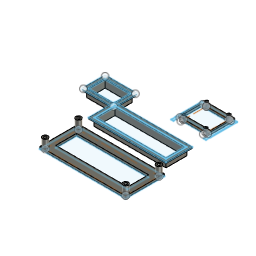
bayesCalc-oled-frame v13 (Autodesk Fusion 360 design; units mm, degrees)
Autodesk Fusion 360 part; units mm, degrees
note: some values were not read from the file. Set by a fixed rule: which sketch regions a step uses.
sketch "Sketch1" plane through (0, 0, 0) normal (0, 0, 1) x (1, 0, 0)
  line L0 (-26.7, -2.5) -> (-1.5, -2.5)
  line L1 (-1.5, -2.5) -> (-1.5, -19.7)
  line L2 (-1.5, -19.7) -> (-26.7, -19.7)
  line L3 (-26.7, -19.7) -> (-26.7, -2.5)
  line L4 (-2.5, -18.7) -> (-25.7, -18.7)
  line L5 (-25.7, -18.7) -> (-25.7, -3.5)
  line L6 (-25.7, -3.5) -> (-2.5, -3.5)
  line L7 (-2.5, -3.5) -> (-2.5, -18.7)
  line L8 (-29.2, -21.2) -> (-29.2, -1)
  line L9 (-28.2, 0) -> (0, 0)
  line L10 (1, -1) -> (1, -21.2)
  line L11 (0, -22.2) -> (-28.2, -22.2)
  arc A0 (1, -1) -> (0, 0) centre (0, -1) ccw
  arc A1 (0, -22.2) -> (1, -21.2) centre (0, -21.2) ccw
  arc A2 (-28.2, 0) -> (-29.2, -1) centre (-28.2, -1) ccw
  arc A3 (-29.2, -21.2) -> (-28.2, -22.2) centre (-28.2, -21.2) ccw
  dimension "d1" = 25.2
  dimension "d2" = 17.2
  dimension "d3" = 1
  dimension "d36" = 1
  dimension "d37" = 1
  dimension "d50" = 2.5
  dimension "d51" = 2.5
  dimension "d52" = 2.5
  dimension "d53" = 2.5
  constraint horizontal L0
  constraint vertical L1
  constraint horizontal L2
  constraint vertical L3
  constraint parallel L3 L8
  constraint parallel L0 L9
  constraint parallel L1 L10
  constraint parallel L2 L11
  constraint tangent L9 A0
  constraint tangent L10 A0
  constraint tangent L10 A1
  constraint tangent L11 A1
  constraint tangent L8 A2
  constraint tangent L9 A2
  constraint equal A1 A2
  constraint tangent L8 A3
  constraint tangent L11 A3
  constraint equal A1 A3
  measures "d1" distance of L0.start L0.end
  measures "d2" distance of L0.start L2.end
  measures "d36" radius of A0
  measures "d37" radius of A1
  measures "d50" distance of L2 L11
  measures "d51" distance of L0 L9
  measures "d52" distance of L3 L8
  measures "d53" distance of L1 L10
extrude "Extrude1" add sketch "Sketch1" against normal blind 7 contours L0 L1 L2 L3 makes body 1
extrude "Extrude2" add sketch "Sketch1" against normal blind 1 separate body contours L8 L9 L10 L11 A0 A1 A2 A3 makes body 2
sketch "Sketch2" plane through (0, 0, 0) normal (0, 0, 1) x (1, 0, 0)
  line L0 (41, 20) -> (66.5, 20)
  line L1 (66.5, 20) -> (66.5, 2.5)
  line L2 (66.5, 2.5) -> (41, 2.5)
  line L3 (41, 2.5) -> (41, 20)
  line L4 (70, -1) -> (37.5, -1)
  line L5 (37.5, -1) -> (37.5, 23.5)
  line L6 (37.5, 23.5) -> (70, 23.5)
  line L7 (70, 23.5) -> (70, -1)
  line L8 (37.5, 23.5) -> (39.5, 23.5)
  line L9 (39.5, 23.5) -> (39.5, -4.9544)
  line L10 (39.5, -4.9544) -> (37.5, -4.9544)
  line L11 (37.5, -4.9544) -> (37.5, 23.5)
  line L12 (70, 23.5) -> (68, 23.5)
  line L13 (68, 23.5) -> (68, -5.1657)
  line L14 (68, -5.1657) -> (70, -5.1657)
  line L15 (70, -5.1657) -> (70, 23.5)
  line L16 (40, 22) -> (66, 22) construction
  line L17 (40, 0.5) -> (65.989, 0.5) construction
  line L18 (43.25, -1.847) -> (43.25, 22.398) construction
  line L19 (64.25, 22.5565) -> (64.25, -1.9527) construction
  circle A0 centre (43.25, 22) radius 1.5
  circle A1 centre (64.25, 22) radius 1.5
  circle A2 centre (64.25, 0.5) radius 1.5
  circle A3 centre (43.25, 0.5) radius 1.5
  circle A4 centre (43.25, 22) radius 0.75
  circle A5 centre (64.25, 22) radius 0.75
  circle A6 centre (43.25, 0.5) radius 0.75
  circle A7 centre (64.25, 0.5) radius 0.75
  dimension "d9" = 25.5
  dimension "d10" = 17.5
  dimension "d11" = -3.5
  dimension "d14" = 2
  dimension "d15" = 2
  dimension "d20" = 2
  dimension "d21" = 2
  dimension "d22" = 2.25
  dimension "d23" = 2.25
  dimension "d24" = 3
  dimension "d25" = 3
  dimension "d26" = 3
  dimension "d27" = 3
  dimension "d38" = 1.5
  dimension "d39" = 1.5
  dimension "d40" = 1.5
  dimension "d41" = 1.5
  constraint horizontal L0
  constraint vertical L1
  constraint horizontal L2
  constraint vertical L3
  constraint horizontal L8
  constraint vertical L9
  constraint horizontal L10
  constraint vertical L11
  constraint horizontal L12
  constraint vertical L13
  constraint horizontal L14
  constraint vertical L15
  constraint perpendicular L13 L16
  constraint perpendicular L13 L17
  constraint perpendicular L16 L18
  constraint perpendicular L17 L19
  constraint coincident L16 A0.centre
  constraint coincident L18 A0.centre
  constraint coincident L16 A1.centre
  constraint coincident L19 A1.centre
  constraint coincident L17 A2.centre
  constraint coincident L19 A2.centre
  constraint coincident L17 A3.centre
  constraint coincident L18 A3.centre
  constraint concentric A0 A4
  constraint concentric A1 A5
  constraint concentric A3 A6
  constraint concentric A2 A7
  measures "d9" distance of L0.start L0.end
  measures "d10" distance of L0.start L2.end
  measures "d14" distance of L5.end L8.end
  measures "d15" distance of L6.end L12.end
  measures "d20" distance of L0 L16
  measures "d21" distance of L2 L17
  measures "d22" distance of L3 L18
  measures "d23" distance of L1 L19
  measures "d24" diameter of A1
  measures "d25" diameter of A0
  measures "d26" diameter of A2
  measures "d27" diameter of A3
  measures "d38" diameter of A4
  measures "d39" diameter of A5
  measures "d40" diameter of A6
  measures "d41" diameter of A7
extrude "Extrude3" add sketch "Sketch2" along normal blind 2 separate body contours L4 L6 L7 L12 L13 L15 | A1 | A0 | A3 | A2 | L4 L6 L9 L13 | L4 L5 L6 L8 L9 L11 | A4 | A5 | A6 | A7 makes body 3
extrude "Extrude4" cut sketch "Sketch2" along normal blind 6 contours L4 L5 L6 L8 L9 L11 bodies 3
extrude "Extrude5" cut sketch "Sketch2" along normal blind 6 contours L4 L13 L14 L15 | L4 L6 L7 L12 L13 L15 bodies 3
extrude "Extrude6" add sketch "Sketch2" along normal blind 4 contours A3 | A6 bodies 3
extrude "Extrude7" add sketch "Sketch2" along normal blind 4 contours A2 | A7 bodies 3
extrude "Extrude8" add sketch "Sketch2" along normal blind 4 contours A0 | A4 bodies 3
extrude "Extrude9" add sketch "Sketch2" along normal blind 4 contours A1 | A5 bodies 3
extrude "Extrude10" cut sketch "Sketch2" along normal blind 4 contours A6 bodies 3
extrude "Extrude11" cut sketch "Sketch2" along normal blind 4 contours A7 bodies 3
extrude "Extrude12" cut sketch "Sketch2" along normal blind 4 contours A4 bodies 3
extrude "Extrude13" cut sketch "Sketch2" along normal blind 4 contours A5 bodies 3
sketch "Sketch3" plane through (0, 0, 0) normal (0, 0, 1) x (1, 0, 0)
  line L0 (0, -20) -> (67, -20)
  line L1 (67, -20) -> (67, -39.5)
  line L2 (67, -39.5) -> (0, -39.5)
  line L3 (0, -39.5) -> (0, -20)
  line L4 (66, -38.5) -> (1, -38.5)
  line L5 (1, -38.5) -> (1, -21)
  line L6 (1, -21) -> (66, -21)
  line L7 (66, -21) -> (66, -38.5)
  line L8 (69.5, -42) -> (-2.5, -42)
  line L9 (-2.5, -42) -> (-2.5, -17.5)
  line L10 (-2.5, -17.5) -> (69.5, -17.5)
  line L11 (69.5, -17.5) -> (69.5, -42)
  dimension "d54" = 67
  dimension "d55" = 19.5
  dimension "d56" = 1
  dimension "d57" = -2.5
  constraint horizontal L0
  constraint vertical L1
  constraint horizontal L2
  constraint vertical L3
  measures "d54" distance of L0.start L0.end
  measures "d55" distance of L0.start L2.end
extrude "Extrude14" add sketch "Sketch3" against normal blind 7 separate body contours L0 L1 L2 L3 makes body 4
extrude "Extrude15" add sketch "Sketch3" against normal blind 1 contours L8 L9 L10 L11 bodies 4
sketch "Sketch5" plane through (0, 0, 0) normal (0, 0, 1) x (1, 0, 0)
  line L0 (0, -90) -> (80, -90)
  line L1 (80, -90) -> (80, -54)
  line L2 (80, -54) -> (0, -54)
  line L3 (0, -54) -> (0, -90)
  line L4 (6.5, -81.75) -> (73.5, -81.75)
  line L5 (73.5, -81.75) -> (73.5, -62.25)
  line L6 (73.5, -62.25) -> (6.5, -62.25)
  line L7 (6.5, -62.25) -> (6.5, -81.75)
  line L8 (0, -87.5) -> (80, -87.5) construction
  line L9 (0, -56.5) -> (80, -56.5) construction
  line L10 (2.5, -90) -> (2.5, -54) construction
  line L11 (77.5, -90) -> (77.5, -54) construction
  circle A0 centre (2.5, -87.5) radius 2.5
  circle A1 centre (77.5, -87.5) radius 2.5
  circle A2 centre (2.5, -56.5) radius 2.5
  circle A3 centre (77.5, -56.5) radius 2.5
  circle A4 centre (2.5, -87.5) radius 1.25
  circle A5 centre (77.5, -87.5) radius 1.25
  circle A6 centre (2.5, -56.5) radius 1.25
  circle A7 centre (77.5, -56.5) radius 1.25
  dimension "d62" = 80
  dimension "d63" = 36
  dimension "d64" = 67
  dimension "d65" = 19.5
  dimension "d66" = 6.5
  dimension "d67" = 8.25
  dimension "d68" = 31
  dimension "d69" = 2.5
  dimension "d70" = 75
  dimension "d71" = 2.5
  dimension "d72" = 5
  dimension "d73" = 5
  dimension "d74" = 5
  dimension "d75" = 5
  dimension "d76" = 2.5
  dimension "d77" = 2.5
  dimension "d78" = 2.5
  dimension "d79" = 2.5
  constraint horizontal L0
  constraint vertical L1
  constraint horizontal L2
  constraint vertical L3
  constraint horizontal L4
  constraint vertical L5
  constraint horizontal L6
  constraint vertical L7
  constraint coincident L3 L8.start
  constraint coincident L1 L8.end
  constraint perpendicular L1 L8
  constraint coincident L3 L9.start
  constraint coincident L1 L9.end
  constraint perpendicular L1 L9
  constraint coincident L0 L10.start
  constraint coincident L2 L10.end
  constraint perpendicular L2 L10
  constraint coincident L0 L11.start
  constraint coincident L2 L11.end
  constraint perpendicular L2 L11
  constraint coincident L10 A0.centre
  constraint coincident L8 A0.centre
  constraint coincident L11 A1.centre
  constraint coincident L8 A1.centre
  constraint coincident L10 A2.centre
  constraint coincident L9 A2.centre
  constraint coincident L11 A3.centre
  constraint coincident L9 A3.centre
  constraint concentric A0 A4
  constraint concentric A1 A5
  constraint concentric A2 A6
  constraint concentric A3 A7
  measures "d62" distance of L0.start L0.end
  measures "d63" distance of L0.start L2.end
  measures "d64" distance of L4.start L4.end
  measures "d65" distance of L4.start L6.end
  measures "d66" distance of L1 L5
  measures "d67" distance of L0 L4
  measures "d68" distance of L8 L9
  measures "d69" distance of L0 L8
  measures "d70" distance of L10 L11
  measures "d71" distance of L3 L10
  measures "d72" diameter of A0
  measures "d73" diameter of A1
  measures "d74" diameter of A2
  measures "d75" diameter of A3
  measures "d76" diameter of A4
  measures "d77" diameter of A5
  measures "d78" diameter of A6
  measures "d79" diameter of A7
extrude "Extrude16" add sketch "Sketch5" along normal blind 2 separate body contours L0 L3 A0 | L0 L1 L2 L3 A0 A1 A2 A3 | L0 L1 A1 | L2 L3 A2 | L1 L2 A3 makes body 5 at (51.1667, -85.7467, 0)
extrude "Extrude17" add sketch "Sketch5" along normal blind 9.5 contours A0 | A1 | A2 | A3 bodies 5
